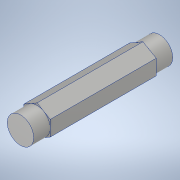
# Autodesk Inventor part: SHAFT
Saved by Autodesk Inventor 2020 (Build 240168000, 168)
## iProperties
RuleStatus: InUse
AfterMaterialChange0: size
AfterDocNew0: SHOW
AfterDocOpen0: SHOW
AfterDocOpen1: size
AfterDocOpen2: DISABLE SHOW
BeforeDocSave0: size
BeforeDocSave1: DISABLE SHOW
AfterDocSave0: DISABLE SHOW
AfterFeatureSuppressionChange0: size
AfterFeatureSuppressionChange1: DISABLE SHOW
PartBodyChanged0: size
PartBodyChanged1: DISABLE SHOW
Created: 2019-04-30
Part Number: SHAFT
Material: Aluminum 6061
Document SubType Name: Modeling
Designer: brand
Density: 2.7 g/cm^3
Appearance: Aluminum - Flat
Mass: 24.5797 g
Surface Area: 31.4663 cm^2
Volume: 9.10358 cm^3
Author: brand
Autodesk Inventor part; units mm, degrees
ref_plane "YZ Plane" through (0, 0, 0) normal (1, 0, 0) x (0, 1, 0)
ref_plane "XZ Plane" through (0, 0, 0) normal (0, 1, 0) x (-1, 0, 0)
ref_plane "XY Plane" through (0, 0, 0) normal (0, 0, 1) x (1, 0, 0)
sketch "Sketch1" plane through (0, 0, 0) normal (0, 0, 1) x (1, 0, 0)
  line L0 (-6.35, -3.6662) -> (-6.35, 3.6662)
  line L1 (-6.35, 3.6662) -> (0, 7.3323)
  line L2 (0, 7.3323) -> (6.35, 3.6662)
  line L3 (6.35, 3.6662) -> (6.35, -3.6662)
  line L4 (6.35, -3.6662) -> (0, -7.3323)
  line L5 (0, -7.3323) -> (-6.35, -3.6662)
  point P0 (0, 0)
  point P1 (0, 0)
  dimension "Size" = 12.7
  constraints: 12 end point, 1 coincident, 1 vertical alignment, 13 other
  measures "Size" distance between parallel lines of L3 L0
extrude "Extrusion1" add sketch "Sketch1" along normal mid plane 50.8
sketch "Sketch2" plane through (0, 0, 25.4) normal (0, 0, 1) x (1, 0, 0)
  line L0 (-6.35, 3.6662) -> (-6.35, -3.6662) construction
  line L1 (-6.35, -3.6662) -> (0, -7.3323) construction
  line L2 (0, -7.3323) -> (6.35, -3.6662) construction
  line L3 (6.35, -3.6662) -> (6.35, 3.6662) construction
  line L4 (6.35, 3.6662) -> (0, 7.3323) construction
  line L5 (0, 7.3323) -> (-6.35, 3.6662) construction
  circle A0 centre (0, 0) radius 6.35
  constraints: 1 centre point, 1 coincident, 1 tangent
extrude "Extrusion2" add sketch "Sketch2" along normal blind 7.9248
mirror "Mirror1" about plane through (0, 0, 0) normal (0, 0, 1) of "Extrusion2"
body "Solid1"
